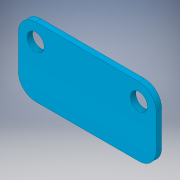
# Autodesk Inventor part: microB
Saved by Autodesk Inventor 2017 (Build 210142000, 142)
## iProperties
Created: 2019-07-28
Part Number: microB
Material: Generic
Document SubType Name: Modeling
Designer: Mitch
Density: 1 g/cm^3
Appearance: Sky Blue Medium
Author: Mitch
Autodesk Inventor part; units mm, degrees
ref_plane "YZ Plane" through (0, 0, 0) normal (1, 0, 0) x (0, 1, 0)
ref_plane "XZ Plane" through (0, 0, 0) normal (0, 1, 0) x (-1, 0, 0)
ref_plane "XY Plane" through (0, 0, 0) normal (0, 0, 1) x (1, 0, 0)
sketch "Sketch1" plane through (0, 0, 0) normal (0, 0, 1) x (1, 0, 0)
  line L0 (2.54, 0) -> (17.78, 0)
  line L1 (20.32, 2.54) -> (20.32, 7.62)
  line L2 (17.78, 10.16) -> (2.54, 10.16)
  line L3 (0, 7.62) -> (0, 2.54)
  arc A0 (2.54, 10.16) -> (0, 7.62) centre (2.54, 7.62) ccw
  arc A1 (20.32, 7.62) -> (17.78, 10.16) centre (17.78, 7.62) ccw
  arc A2 (17.78, 0) -> (20.32, 2.54) centre (17.78, 2.54) ccw
  arc A3 (0, 2.54) -> (2.54, 0) centre (2.54, 2.54) ccw
  circle A4 centre (2.54, 7.62) radius 1.27
  circle A5 centre (17.78, 7.62) radius 1.27
  point P0 (0, 0)
  point P1 (20.32, 10.16)
  point P2 (20.32, 0)
  point P3 (0, 10.16)
  dimension "d0" = 20.32
  dimension "d1" = 10.16
  dimension "d2" = 2.54
  dimension "d3" = 2.54
  dimension "d4" = 2.54
  dimension "d5" = 2.54
  dimension "d6" = 2.54
  dimension "d7" = 15.24
  constraints: 8 end point, 8 point on circle, 8 point on line, 8 tangent, 6 centre point, 3 equal radius, 2 parallel, 1 horizontal, 1 perpendicular
  measures "d0" distance of point (0, 10.16) point (20.32, 10.16)
  measures "d1" distance of point (20.32, 10.16) point (20.32, 0)
  measures "d2" radius of A0
  measures "d3" diameter of A4
  measures "d4" distance from line of L3 A4.centre
  measures "d5" distance from line of L2 A4.centre
  measures "d6" diameter of A5
  measures "d7" distance of A4.centre A5.centre
extrude "Extrusion1" add sketch "Sketch1" along normal blind 0.8128
body "Solid1"
